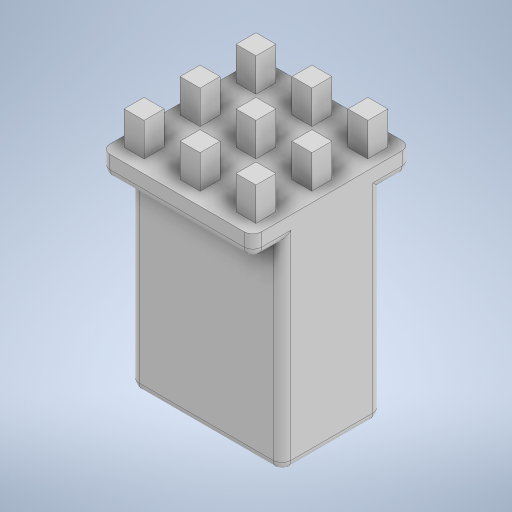
# Autodesk Inventor part: Platform
Saved by Autodesk Inventor 2024.1 (Build 281209000, 209)
## iProperties
Created: 2024-04-30
Part Number: Platform
Material: Generic
Document SubType Name: Modeling
Designer: cyan924
Density: 1 g/cm^3
Appearance: Default
Author: cyan924
Autodesk Inventor part; units mm, degrees
ref_plane "YZ Plane" through (0, 0, 0) normal (1, 0, 0) x (0, 1, 0)
ref_plane "XZ Plane" through (0, 0, 0) normal (0, 1, 0) x (-1, 0, 0)
ref_plane "XY Plane" through (0, 0, 0) normal (0, 0, 1) x (1, 0, 0)
sketch "Sketch1" plane through (0, 0, 0) normal (0, 1, 0) x (-1, 0, 0)
  line L0 (0, 0) -> (34.2, 0)
  line L1 (34.2, 0) -> (34.2, -22.5)
  line L2 (34.2, -22.5) -> (0, -22.5)
  line L3 (0, -22.5) -> (0, 0)
  line L4 (5, -17.5) -> (29.2, -17.5)
  line L5 (29.2, -17.5) -> (29.2, -5)
  line L6 (29.2, -5) -> (5, -5)
  line L7 (5, -5) -> (5, -17.5)
  dimension "d64" = 24.2
  dimension "d65" = 12.5
  dimension "d66" = 5
  dimension "d67" = 5
  dimension "d68" = 5
  dimension "d69" = 5
  constraints: 16 end point, 4 parallel, 2 horizontal, 2 perpendicular
  measures "d64" distance between parallel lines of L5 L7
  measures "d65" distance of L4.end L5.end
  measures "d66" distance between parallel lines of L1 L5
  measures "d67" distance between parallel lines of L3 L7
  measures "d68" distance between parallel lines of L0 L6
  measures "d69" distance between parallel lines of L2 L4
extrude "Extrusion4" add sketch "Sketch1" along normal blind 16.4
sketch "Sketch6" plane through (0, 16.4, 0) normal (0, 1, 0) x (1, 0, 0)
  line L0 (-34.2, 0) -> (0, 0) projected
  line L1 (0, 22.5) -> (-34.2, 22.5) projected
  line L2 (-34.2, 0) -> (0, 0)
  line L3 (0, 0) -> (0, 22.5)
  line L4 (0, 22.5) -> (-34.2, 22.5)
  line L5 (-34.2, 22.5) -> (-34.2, 0)
  constraints: 8 end point, 2 parallel, 1 horizontal, 1 perpendicular
extrude "Extrusion6" add sketch "Sketch6" along normal blind 33.5
sketch "Sketch8" plane through (-34.2, 0, -22.5) normal (-1, 0, 0) x (0, 0, 1)
  line L0 (17.5, 0) -> (17.5, 16.4) projected
  line L1 (5, 16.4) -> (17.5, 16.4) projected
  line L2 (17.5, 6.4) -> (5, 6.4)
  line L3 (5, 6.4) -> (5, 16.4)
  line L4 (5, 16.4) -> (17.5, 16.4)
  line L5 (17.5, 16.4) -> (17.5, 6.4)
  point P0 (22.5, 0)
  dimension "d176" = 10
  constraints: 8 end point, 2 parallel, 1 horizontal, 1 perpendicular, 1 point on line
  measures "d176" distance between parallel lines of L1 L2
extrude "Extrusion8" cut sketch "Sketch8" against normal blind 7.5
fillet "Fillet2" radius 2 11 edges at (-17.1, 0, -22.5) (-34.2, 0, -11.25) (0, 0, -11.25) (-17.1, 0, 0) (0, 24.95, -22.5) (0, 24.95, 0) (-34.2, 24.95, -22.5) (-34.2, 24.95, 0) (-34.2, 11.4, -5) (-34.2, 6.4, -11.25) (-34.2, 11.4, -17.5)
sketch "Sketch9" plane through (0, 49.9, 0) normal (0, 1, 0) x (1, 0, 0)
  line L0 (-34.2, 11.25) -> (0, 11.25) construction
  line L1 (0, 20.5) -> (0, 2) construction
  line L2 (-32.2, 22.5) -> (-2, 22.5) construction
  line L3 (-17.1, 22.5) -> (-17.1, 0) construction
  line L4 (-32.2, 0) -> (-2, 0) construction
  line L5 (-17.1, 11.25) -> (-17.1, 13.5) construction
  line L6 (-17.1, 13.5) -> (-14.85, 13.5) construction
  line L7 (-14.85, 13.5) -> (-19.35, 13.5)
  line L8 (-19.35, 13.5) -> (-19.35, 9)
  line L9 (-19.35, 9) -> (-14.85, 9)
  line L10 (-14.85, 9) -> (-14.85, 13.5)
  line L11 (-19.35, 11.25) -> (-27.45, 11.25) construction
  line L12 (-27.45, 11.25) -> (-27.45, 13.5) construction
  line L13 (-27.45, 13.5) -> (-31.95, 13.5)
  line L14 (-31.95, 13.5) -> (-31.95, 9)
  line L15 (-31.95, 9) -> (-27.45, 9)
  line L16 (-27.45, 9) -> (-27.45, 13.5)
  line L17 (-14.85, 11.25) -> (-6.75, 11.25) construction
  line L18 (-6.75, 11.25) -> (-6.75, 13.5) construction
  line L19 (-6.75, 13.5) -> (-2.25, 13.5)
  line L20 (-2.25, 13.5) -> (-2.25, 9)
  line L21 (-2.25, 9) -> (-6.75, 9)
  line L22 (-6.75, 9) -> (-6.75, 13.5)
  line L23 (-31.95, 13.5) -> (-31.95, 21.6) construction
  line L24 (-31.95, 21.6) -> (-27.45, 21.6)
  line L25 (-27.45, 21.6) -> (-27.45, 26.1)
  line L26 (-27.45, 26.1) -> (-31.95, 26.1)
  line L27 (-31.95, 26.1) -> (-31.95, 21.6)
  line L28 (-19.35, 13.5) -> (-19.35, 21.6) construction
  line L29 (-6.75, 13.5) -> (-6.75, 21.6) construction
  line L30 (-31.95, 9) -> (-31.95, 0.9) construction
  line L31 (-19.35, 9) -> (-19.35, 0.9) construction
  line L32 (-6.75, 9) -> (-6.75, 0.9) construction
  line L33 (-19.35, 21.6) -> (-14.85, 21.6)
  line L34 (-14.85, 21.6) -> (-14.85, 26.1)
  line L35 (-14.85, 26.1) -> (-19.35, 26.1)
  line L36 (-19.35, 26.1) -> (-19.35, 21.6)
  line L37 (-6.75, 21.6) -> (-2.25, 21.6)
  line L38 (-2.25, 21.6) -> (-2.25, 26.1)
  line L39 (-2.25, 26.1) -> (-6.75, 26.1)
  line L40 (-6.75, 26.1) -> (-6.75, 21.6)
  line L41 (-6.75, 0.9) -> (-2.25, 0.9)
  line L42 (-2.25, 0.9) -> (-2.25, -3.6)
  line L43 (-2.25, -3.6) -> (-6.75, -3.6)
  line L44 (-6.75, -3.6) -> (-6.75, 0.9)
  line L45 (-19.35, 0.9) -> (-14.85, 0.9)
  line L46 (-14.85, 0.9) -> (-14.85, -3.6)
  line L47 (-14.85, -3.6) -> (-19.35, -3.6)
  line L48 (-19.35, -3.6) -> (-19.35, 0.9)
  line L49 (-31.95, 0.9) -> (-27.45, 0.9)
  line L50 (-27.45, 0.9) -> (-27.45, -3.6)
  line L51 (-27.45, -3.6) -> (-31.95, -3.6)
  line L52 (-31.95, -3.6) -> (-31.95, 0.9)
  dimension "d202" = 2.25
  dimension "d203" = 2.25
  dimension "d204" = 4.5
  dimension "d205" = 4.5
  dimension "d206" = 8.1
  dimension "d207" = 2.25
  dimension "d208" = 4.5
  dimension "d209" = 4.5
  dimension "d210" = 8.1
  dimension "d211" = 2.25
  dimension "d212" = 4.5
  dimension "d213" = 4.5
  dimension "d214" = 8.1
  dimension "d215" = 4.5
  dimension "d216" = 4.5
  dimension "d217" = 8.1
  dimension "d218" = 8.1
  dimension "d219" = 8.1
  dimension "d220" = 90
  dimension "d221" = 8.1
  dimension "d222" = 8.1
  dimension "d223" = 4.5
  dimension "d224" = 4.5
  dimension "d225" = 4.5
  dimension "d226" = 4.5
  dimension "d227" = 4.5
  dimension "d228" = 4.5
  dimension "d229" = 4.5
  dimension "d230" = 4.5
  dimension "d231" = 4.5
  dimension "d232" = 4.5
  constraints: 100 end point, 18 parallel, 13 perpendicular, 9 horizontal, 6 midpoint, 4 point on line, 3 vertical
  measures "d202" distance of L5.start L5.end
  measures "d203" distance of L5.end L6.end
  measures "d204" distance of L9.end L8.end
  measures "d205" distance of L8.end L7.end
  measures "d206" distance of L11.start L11.end
  measures "d207" distance of L11.end L12.end
  measures "d208" distance of L15.end L14.end
  measures "d209" distance of L14.end L13.end
  measures "d210" distance of L17.start L17.end
  measures "d211" distance of L17.end L18.end
  measures "d212" distance of L20.end L21.end
  measures "d213" distance of L19.end L20.end
  measures "d214" distance of L13.end L23.end
  measures "d215" distance of L26.end L25.end
  measures "d216" distance of L25.end L24.end
  measures "d217" distance of L7.end L28.end
  measures "d218" distance of L18.end L29.end
  measures "d219" distance of L14.end L30.end
  measures "d220" angle of L15 L30
  measures "d221" distance of L8.end L31.end
  measures "d222" distance of L21.end L32.end
  measures "d223" distance of L35.end L34.end
  measures "d224" distance of L34.end L33.end
  measures "d225" distance of L39.end L38.end
  measures "d226" distance of L38.end L37.end
  measures "d227" distance of L42.end L43.end
  measures "d228" distance of L41.end L42.end
  measures "d229" distance of L46.end L47.end
  measures "d230" distance of L45.end L46.end
  measures "d231" distance of L50.end L51.end
  measures "d232" distance of L49.end L50.end
extrude "Extrusion9" add sketch "Sketch9" along normal blind 7.5
sketch "Sketch10" plane through (0, 49.9, 0) normal (0, 1, 0) x (1, 0, 0)
  line L0 (0, 2) -> (0, 20.5) construction
  line L1 (0, 20.5) -> (0, 29.05) construction
  line L2 (-34.2, 20.5) -> (-34.2, 2) construction
  line L3 (-34.2, 2) -> (-34.2, -6.55) construction
  line L4 (0, 29.05) -> (-34.2, 29.05)
  line L5 (-34.2, 29.05) -> (-34.2, -6.55)
  line L6 (-34.2, -6.55) -> (0, -6.55)
  line L7 (0, -6.55) -> (0, 29.05)
  point P0 (0, 0)
  dimension "d233" = 8.55
  dimension "d234" = 8.55
  constraints: 12 end point, 2 parallel, 2 vertical, 1 horizontal, 1 perpendicular
  measures "d233" distance of L0.end L1.end
  measures "d234" distance of L2.end L3.end
extrude "Extrusion10" add sketch "Sketch10" against normal blind 5
fillet "Fillet3" radius 2 10 edges at (-34.2, 44.9, -24.775) (-17.1, 44.9, -29.05) (-34.2, 47.4, 6.55) (-34.2, 44.9, 2.275) (-17.1, 44.9, 6.55) (0, 44.9, 2.275) (0, 47.4, 6.55) (0, 44.9, -24.775) (0, 47.4, -29.05) (-34.2, 47.4, -29.05)
equation "\"box\" = 4.5"
equation "\"walllength\" = 1"
equation "\"gap\" = 8.1"
equation "\"d34\" = 4.6"
equation "\"d35\" = 8"
equation "\"offset\" = 5"
equation "\"d44\" = 4.6"
equation "\"d89\" = 4.6"
equation "\"d126\" = 4.6"
equation "\"d134\" = 4.6"
equation "\"d135\" = 8"
equation "\"d140\" = 4.6"
equation "\"d144\" = 4.6"
equation "\"d162\" = 4.6"
equation "\"d163\" = 4.6"
equation "\"d164\" = 8"
equation "\"d165\" = 4.6"
equation "\"d166\" = 4.6"
equation "\"d167\" = 4.6"
body "Solid2"
